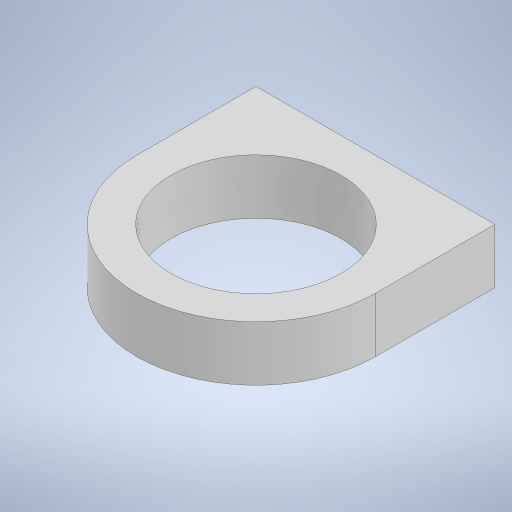
# Autodesk Inventor part: borde al borde chico
Saved by Autodesk Inventor 2024 (Build 280153000, 153)
## iProperties
Created: 2024-04-11
Part Number: borde al borde chico
Material: Generic
Document SubType Name: Modeling
Designer: compu
Density: 1 g/cm^3
Appearance: Default
Author: compu
Autodesk Inventor part; units mm, degrees
ref_plane "YZ Plane" through (0, 0, 0) normal (1, 0, 0) x (0, 1, 0)
ref_plane "XZ Plane" through (0, 0, 0) normal (0, 1, 0) x (-1, 0, 0)
ref_plane "XY Plane" through (0, 0, 0) normal (0, 0, 1) x (1, 0, 0)
sketch "Sketch1" plane through (0, 0, 0) normal (0, 1, 0) x (-1, 0, 0)
  circle A0 centre (0, 0) radius 2
  circle A1 centre (0, 0) radius 6.2
  circle A2 centre (0, 0) radius 8.7
  line L0 (12.18, 0) -> (-12.18, 0) projected
  line L1 (0, -12.18) -> (0, 12.18) projected
  line L2 (8.7, 0) -> (8.7, -8.7)
  line L3 (8.7, -8.7) -> (-8.7, -8.7)
  line L4 (-8.7, -8.7) -> (-8.7, 0)
  dimension "d0" = 4
  dimension "d1" = 12.4
  dimension "d2" = 17.4
  dimension "d3" = 17.4
  constraints: 6 end point, 3 centre point, 3 coincident, 2 point on circle, 2 tangent, 1 parallel, 1 perpendicular, 1 point on line
  measures "d0" diameter of A0
  measures "d1" diameter of A1
  measures "d2" diameter of A2
  measures "d3" distance of L2.end L3.end
extrude "Extrusion1" add sketch "Sketch1" along normal blind 4 contours L0 A2 L1 A1 | A1 L1 A2 L0 | A1 L0 A2 L1 | L1 A2 L0 A1 | L2 L3 A2 | L3 L4 A2
body "Solid1"
